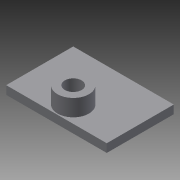
# Autodesk Inventor part: fijador.rodamiento
Saved by Autodesk Inventor 2015 SP1 (Build 190203100, 203)
## iProperties
Created: 2015-06-17
Part Number: fijador.rodamiento
Material: Generic
Document SubType Name: Modeling
Designer: pc
Density: 1 g/cm^3
Appearance: Default
Author: pc
Autodesk Inventor part; units mm, degrees
ref_plane "YZ Plane" through (0, 0, 0) normal (1, 0, 0) x (0, 1, 0)
ref_plane "XZ Plane" through (0, 0, 0) normal (0, 1, 0) x (-1, 0, 0)
ref_plane "XY Plane" through (0, 0, 0) normal (0, 0, 1) x (1, 0, 0)
sketch "Sketch2" plane through (0, 0, 0) normal (0, 0, 1) x (1, 0, 0)
  circle A0 centre (0, 0) radius 3.75
  circle A1 centre (0, 0) radius 2
  dimension "d6" = 7.5
  dimension "d7" = 4
  constraints: 2 centre point, 2 coincident
  measures "d6" diameter of A0
  measures "d7" diameter of A1
extrude "Extrusion1" add sketch "Sketch2" along normal blind 6
sketch "Sketch3" plane through (0, 0, 0) normal (0, 0, -1) x (-1, 0, 0)
  line L0 (-12, -4) -> (12, -4)
  line L1 (12, -4) -> (12, 12)
  line L2 (12, 12) -> (-12, 12)
  line L3 (-12, 12) -> (-12, -4)
  line L4 (0, 0) -> (0, 4.4651)
  line L5 (0, 4.4651) -> (0, 0)
  line L6 (0, 0) -> (5, 0)
  circle A0 centre (0, 0) radius 2 projected
  circle A1 centre (0, 0) radius 2
  dimension "d10" = 24
  dimension "d11" = 16
  dimension "d12" = 4
  constraints: 14 end point, 3 equal length, 1 centre point, 1 coincident, 1 horizontal, 1 perpendicular, 1 symmetric about line, 1 vertical
  measures "d10" distance of L1.end L2.end
  measures "d11" distance of L2.end L0.start
  measures "d12" distance from line of L0 L4.start
extrude "Extrusion4" add sketch "Sketch3" against normal blind 2
body "Solid2"
